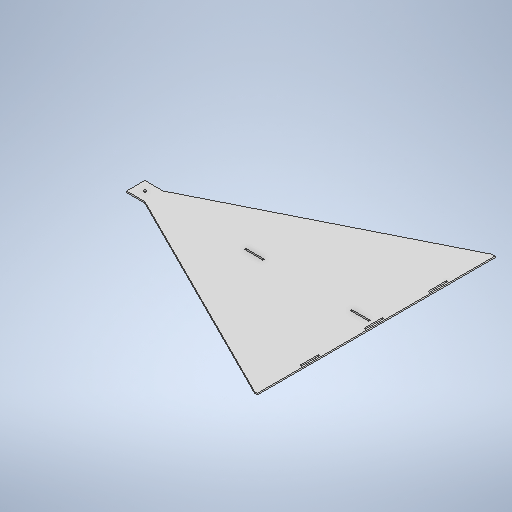
# Autodesk Inventor part: Trebuchet V1 - Truss
Saved by Autodesk Inventor 2025.2 (Build 292293000, 293)
## iProperties
Created: 2025-04-06
Part Number: Trebuchet V1 - Truss
Material: Generic
Document SubType Name: Modeling
Designer: Dylan
Density: 1 g/cm^3
Appearance: Default
Author: VRK99-0110
Title: Trebuchet - Truss
Subject: Trebuchet Project
Autodesk Inventor part; units mm, degrees
ref_plane "YZ Plane" through (0, 0, 0) normal (1, 0, 0) x (0, 1, 0)
ref_plane "XZ Plane" through (0, 0, 0) normal (0, 1, 0) x (-1, 0, 0)
ref_plane "XY Plane" through (0, 0, 0) normal (0, 0, 1) x (1, 0, 0)
sketch "Sketch1" plane through (0, 0, 0) normal (0, 1, 0) x (-1, 0, 0)
  line L0 (0, 260) -> (0, -260)
  line L1 (520, 0) -> (0, 260)
  line L2 (0, -260) -> (520, 0)
  point P0 (0, 0)
  dimension "d1" = 260
  dimension "d2" = 520
  constraints: 6 end point
  measures "d1" distance of point (0, 0) L0.start
  measures "d2" distance of L0.start L0.end
extrude "Extrusion1" add sketch "Sketch1" along normal blind 3.175
sketch "Sketch2" plane through (0, 3.175, 0) normal (0, 1, 0) x (1, 0, 0)
  circle A0 centre (-500, 0) radius 3.175
  point P0 (0, 0)
  dimension "d6" = 6.35
  constraints: 1 centre point
  measures "d6" diameter of A0
extrude "Extrusion2" cut sketch "Sketch2" against normal blind 3.175
sketch "Sketch3" plane through (0, 3.175, 0) normal (0, 1, 0) x (1, 0, 0)
  circle A0 centre (-500, 0) radius 3.175 projected
  line L0 (-500, 0) -> (-480, 0)
  line L1 (-480, 0) -> (-480, -20)
  line L2 (-480, -20) -> (-480, 20)
  line L3 (0, 260) -> (-520, 0) projected
  line L4 (-480, 20) -> (-520, 0)
  line L5 (-520, 0) -> (-480, -20)
  line L6 (-520, 0) -> (0, -260) projected
  point P0 (0, 0)
  constraints: 10 end point, 2 collinear, 1 horizontal, 1 perpendicular, 1 point on line
extrude "Extrusion3" cut sketch "Sketch3" against normal blind 3.175
sketch "Sketch4" plane through (0, 3.175, 0) normal (0, 1, 0) x (1, 0, 0)
  line L0 (-480, -20) -> (-480, 20) projected
  line L1 (-480, -20) -> (-520, -20)
  line L2 (-520, -20) -> (-520, 20)
  line L3 (-520, 20) -> (-480, 20)
  point P0 (0, 0)
  dimension "d11" = 40
  constraints: 6 end point, 2 perpendicular, 1 horizontal
  measures "d11" distance of L0.start L1.end
extrude "Extrusion4" add sketch "Sketch4" against normal blind 3.175
sketch "Sketch5" plane through (0, 3.175, 0) normal (0, 1, 0) x (1, 0, 0)
  circle A0 centre (-500, 0) radius 3.175
  point P0 (0, 0)
  dimension "d15" = 6.35
  constraints: 1 centre point
  measures "d15" diameter of A0
extrude "Extrusion5" cut sketch "Sketch5" against normal blind 3.175
sketch "Sketch6" plane through (0, 3.175, 0) normal (0, 1, 0) x (1, 0, 0)
  line L0 (-480, -20) -> (0, -260) projected
  line L1 (0, -260) -> (50, -260)
  line L2 (50, -260) -> (50, 260)
  line L3 (50, 260) -> (0, 260)
  line L4 (0, 260) -> (0, -260)
  point P0 (0, 0)
  constraints: 8 end point, 3 perpendicular, 1 horizontal
extrude "Extrusion6" add sketch "Sketch6" against normal blind 3.175
sketch "Sketch8" plane through (0, 3.175, 0) normal (0, 1, 0) x (1, 0, 0)
  line L0 (0, 260) -> (-480, 20) projected
  line L1 (-480, -20) -> (0, -260) projected
  line L2 (3.175, -20) -> (0, -20)
  line L3 (0, -20) -> (0, 20)
  line L4 (0, -20) -> (3.2, -20)
  line L5 (0, 20) -> (3.2, 20)
  line L6 (3.2, 20) -> (3.2, -20)
  line L7 (3.2, 160) -> (3.2, 120)
  line L8 (3.2, 120) -> (0, 120)
  line L9 (0, 120) -> (0, 160)
  line L10 (0, 160) -> (3.2, 160)
  line L11 (3.2, -160) -> (3.2, -120)
  line L12 (3.2, -120) -> (0, -120)
  line L13 (0, -120) -> (0, -160)
  line L14 (0, -160) -> (3.2, -160)
  point P0 (0, 0)
  dimension "d23" = 3.2
  dimension "d24" = 3.2
  dimension "d27" = 40
  constraints: 26 end point, 3 horizontal, 3 perpendicular, 1 point on line
  measures "d23" distance of L2.end L4.end
  measures "d24" distance of L3.end L5.end
  measures "d27" distance of L7.start L7.end
extrude "Extrusion7" cut sketch "Sketch8" against normal blind 10
sketch "Sketch9" plane through (0, 3.175, 0) normal (0, 1, 0) x (1, 0, 0)
  line L0 (3.2, -120) -> (3.2, -160) projected
  line L1 (6.4, -260) -> (6.4, 260)
  line L2 (0, 260) -> (50, 260) projected
  line L3 (6.4, 260) -> (50, 260)
  line L4 (50, 260) -> (50, -260)
  line L5 (50, -260) -> (6.4, -260)
  point P0 (0, 0)
  constraints: 8 end point, 1 horizontal, 1 perpendicular, 1 point on line, 1 vertical
extrude "Extrusion8" cut sketch "Sketch9" against normal blind 10
sketch "Sketch10" plane through (0, 3.175, 0) normal (0, 1, 0) x (1, 0, 0)
  line L0 (-520, 20) -> (-520, -20) projected
  line L1 (-240, 1.6) -> (-280, 1.6)
  line L2 (-280, 1.6) -> (-280, -1.6)
  line L3 (-280, -1.6) -> (-240, -1.6)
  line L4 (-240, -1.6) -> (-240, 1.6)
  point P0 (0, 0)
  dimension "d38" = 40
  dimension "d39" = 40
  constraints: 8 end point, 2 perpendicular
  measures "d38" distance of L1.start L1.end
  measures "d39" distance of L2.end L3.end
extrude "Extrusion9" cut sketch "Sketch10" against normal blind 10
sketch "Sketch11" plane through (0, 3.175, 0) normal (0, 1, 0) x (1, 0, 0)
  line L0 (6.4, 260) -> (6.4, -260) projected
  line L1 (-8.6, 1.6) -> (-8.6, -1.6)
  line L2 (-8.6, -1.6) -> (-48.6, -1.6)
  line L3 (-48.6, -1.6) -> (-48.6, 1.6)
  line L4 (-48.6, 1.6) -> (-8.6, 1.6)
  point P0 (0, 0)
  dimension "d44" = 40
  constraints: 8 end point, 2 perpendicular, 1 horizontal
  measures "d44" distance of L1.end L2.end
extrude "Extrusion10" cut sketch "Sketch11" against normal blind 10
body "Solid1"
